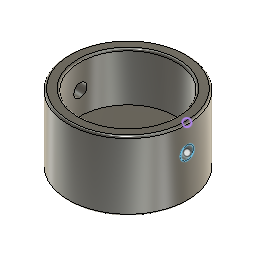
celestron foot (Autodesk Fusion 360 design; units mm, degrees)
Autodesk Fusion 360 part; units mm, degrees
sketch "Base" plane through (0, 0, 0) normal (0, 0, 1) x (1, 0, 0)
  circle A0 centre (0, 0) radius 12.875
  circle A1 centre (0, 0) radius 15.875
  circle A2 centre (0, 0) radius 5.0125
  line L0 (-4.1244, 7.1438) -> (-8.2489, 0) construction
  line L1 (-8.2489, 0) -> (-4.1244, -7.1437) construction
  line L2 (-4.1244, -7.1437) -> (4.1244, -7.1438) construction
  line L3 (4.1244, -7.1438) -> (8.2489, 0) construction
  line L4 (8.2489, 0) -> (4.1244, 7.1437) construction
  line L5 (4.1244, 7.1437) -> (-4.1244, 7.1438) construction
  dimension "d1" = 25.75
  dimension "d2" = 3
  dimension "d3" = 10.025
  dimension "d4" = 7.1437
  constraint coincident A0.centre A1.centre
  constraint concentric A0 A2
  measures "d1" diameter of A0
  measures "d3" diameter of A2
  measures "d4" distance of A0.centre L5
extrude "Extrude1" add sketch "Base" along normal blind 5.5 contours A0
extrude "Extrude2" add sketch "Base" along normal blind 18.5 contours A1
fillet "Fillet1" radius 0.5 2 edges at (-14.8007, -5.7406, 18.5) (-12.0037, 4.6558, 18.5)
fillet "Fillet2" radius 0.5 1 edges at (-14.8007, -5.7406, 0)
ref_plane "WorkPlane1" through (15.8749, -0.0653, 6.6157) normal (0.999992, -0.004114, 0) x (-0.004114, -0.999992, 0)
sketch "Screw Holes" plane through (15.8749, -0.0653, 6.6157) normal (0.999992, -0.004114, 0) x (-0.004114, -0.999992, 0)
  circle A0 centre (0, -4.8993) radius 1.75
  point P0 (0.0633, -11.8843)
  dimension "d12" = 3.5
  dimension "d13" = 6.985
  measures "d12" diameter of A0
  measures "d13" vertical distance of A0.centre P0
extrude "Extrude3" cut sketch "Screw Holes" against normal blind 35
equation "d3 = 0.375 * 1 in + 0.5 mm"
equation "d4 = ( 9 / 16 ) * 1 in / 2"
equation "d13 = 0.275 * 1 in"
